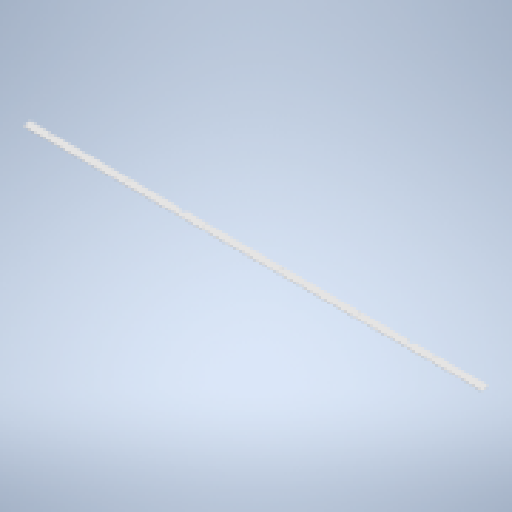
# Autodesk Inventor part: BSH 032 stringer floor 2
Saved by Autodesk Inventor 2025 (Build 290162010, 162A)
## iProperties
Created: 2024-07-23
Part Number: BSH 032 stringer floor 2
Material: 09g2s
Document SubType Name: Sheet Metal
Designer: pokla
Mass: 5330.4 g
Surface Area: 4696.25 cm^2
Volume: 679.031 cm^3
Density: 7.85 g/cm^3
Flat Pattern Width: 298 cm
Flat Pattern Length: 5 cm
Flat Pattern Area: 1490 cm^2
Sheet Metal Rule: AISI304 3mm Die 32
Sheet Metal Width: 2980,000 mm
Sheet Metal Length: 50,000 mm
Sheet Metal Area: 149000,000 mm^2
Appearance: Default
Stock Number: БШК 032 стрингер пол 2
Author: admin
Autodesk Inventor part; units mm, degrees
ref_plane "YZ Plane" through (0, 0, 0) normal (1, 0, 0) x (0, 1, 0)
ref_plane "XZ Plane" through (0, 0, 0) normal (0, 1, 0) x (-1, 0, 0)
ref_plane "XY Plane" through (0, 0, 0) normal (0, 0, 1) x (1, 0, 0)
sketch "Sketch8" plane through (0, 0, 0) normal (0, 0, 1) x (1, 0, 0)
  line L0 (-1490, 50) -> (1490, 50)
  line L1 (1490, 50) -> (1490, 0)
  line L2 (1490, 0) -> (-1490, 0)
  line L3 (-1490, 0) -> (-1490, 50)
  point P0 (0, 0)
  point P1 (0, 0)
  dimension "d37" = 50
  dimension "d38" = 2980
  measures "d37" distance of L0.end L1.end
  measures "d38" distance of L0.start L0.end
extrude "Plate5" add sketch "Sketch8" against normal blind 3
sketch "Sketch9" plane through (0, 0, 0) normal (0, 0, 1) x (1, 0, 0)
  line L0 (1490, 50) -> (-1490, 50) projected
  line L1 (-1197, 50) -> (-1193.8, 50)
  line L2 (-1193.8, 50) -> (-1193.8, 24)
  line L3 (-1193.8, 24) -> (-1197, 24)
  line L4 (-1197, 24) -> (-1197, 50)
  line L5 (-1490, 50) -> (-1490, 0) projected
  point P0 (0, 0)
  point P1 (-1193.8, 50)
  dimension "d42" = 293
  dimension "d43" = 3.2
  dimension "d44" = 26
  constraints: 8 end point, 2 parallel, 1 horizontal, 1 perpendicular, 1 point on line
  measures "d42" distance between parallel lines of L4 L5
  measures "d43" distance between parallel lines of L4 L2
  measures "d44" distance of L1.end L2.end
extrude "Extrusion3" cut sketch "Sketch9" against normal through all
pattern_linear "Rectangular Pattern2" count 6 spacing 500 along (1, 0, 0) of "Extrusion3"
sketch "Sketch10" plane through (0, 0, 0) normal (0, 0, 1) x (1, 0, 0)
  line L0 (1303, 24) -> (1303, 50) projected
  line L1 (1303, 50) -> (806.2, 50) projected
  line L2 (806.2, 50) -> (806.2, 24) projected
  line L3 (806.2, 24) -> (803, 24) projected
  line L4 (803, 24) -> (803, 50) projected
  line L5 (803, 50) -> (306.2, 50) projected
  line L6 (306.2, 50) -> (306.2, 24) projected
  line L7 (306.2, 24) -> (303, 24) projected
  line L8 (303, 24) -> (303, 50) projected
  line L9 (303, 50) -> (-193.8, 50) projected
  line L10 (-193.8, 50) -> (-193.8, 24) projected
  line L11 (-193.8, 24) -> (-197, 24) projected
  line L12 (-197, 24) -> (-197, 50) projected
  line L13 (-197, 50) -> (-693.8, 50) projected
  line L14 (-693.8, 50) -> (-693.8, 24) projected
  line L15 (-693.8, 24) -> (-697, 24) projected
  line L16 (-697, 24) -> (-697, 50) projected
  line L17 (-697, 50) -> (-1193.8, 50) projected
  line L18 (-1193.8, 50) -> (-1193.8, 24) projected
  line L19 (-1193.8, 24) -> (-1197, 24) projected
  line L20 (-1197, 24) -> (-1197, 50) projected
  line L21 (-1197, 50) -> (-1490, 50) projected
  line L22 (-1490, 50) -> (-1490, 0) projected
  line L23 (-1490, 0) -> (1490, 0) projected
  line L24 (1490, 0) -> (1490, 50) projected
  line L25 (1490, 50) -> (1306.2, 50) projected
  line L26 (1306.2, 50) -> (1306.2, 24) projected
  line L27 (1306.2, 24) -> (1303, 24) projected
  circle A0 centre (-490, 50) radius 20
  circle A1 centre (990, 50) radius 20
  point P0 (0, 0)
  point P1 (1340, 50)
  point P2 (1380, 50)
  point P3 (-140, 50)
  point P4 (-100, 50)
  point P5 (970, 50)
  point P6 (1010, 50)
  point P7 (-510, 50)
  point P8 (-470, 50)
  dimension "d50" = 40
  dimension "d51" = 1480
  dimension "d52" = 1000
  constraints: 3 point on line, 2 centre point, 1 equal radius
  measures "d50" diameter of A0
  measures "d51" distance of A0.centre A1.centre
  measures "d52" distance from line of L22 A0.centre
extrude "Extrusion4" cut sketch "Sketch10" against normal through all contours A1 L1 | L1 A1 | A0 L13 | L13 A0
sketch "Sketch11" plane through (0, 0, 0) normal (0, 0, 1) x (1, 0, 0)
  line L0 (-1473.7105, 19.3646) -> (-1242.1993, 19.3646) construction
  line L1 (-1242.1993, 19.3646) -> (-1242.1993, 3.0803) construction
  line L2 (-1242.1993, 3.0803) -> (-1473.7105, 3.0803) construction
  line L3 (-1473.7105, 3.0803) -> (-1473.7105, 19.3646) construction
  point P0 (0, 0)
  constraints: 2 other
mark "Mark1"
equation "\"d41\" = Thickness"
equation "\"BendReliefWidth\" = Thickness"
equation "\"BendReliefDepth\" = 0.5 * Thickness"
equation "\"CornerReliefSize\" = 4 * Thickness"
equation "\"MinimumRemnant\" = 2 * Thickness"
equation "\"TransitionRadius\" = BendRadius"
equation "\"JacobiRadiusSize\" = BendRadius"
equation "\"GapSize\" = Thickness"
equation "\"Thickness\" = 3"
equation "\"BendRadius\" = 5"
body "Solid3"
